Autodesk Fusion 360 part; units mm, degrees
(part 3 of 4)
  spline S294 degree 3 poles (-68.0103, -62.366) (-67.2714, -61.5215) (-66.1636, -61.0119) (-65.0416, -61.0002) (-63.8919, -60.9883) (-62.7469, -61.5006) (-61.9897, -62.366) knots -1 -1 -1 -1 -0.506107 -0.506107 -0.506107 0 0 0 0
  spline S295 degree 3 poles (-61.9897, -62.366) (-61.3663, -63.0785) (-61.0085, -64.0182) (-61.0002, -64.9649) (-60.9916, -65.935) (-61.3508, -66.9039) (-61.9897, -67.634) knots -1 -1 -1 -1 -0.506107 -0.506107 -0.506107 0 0 0 0
  spline S296 degree 3 poles (-61.9897, -57.634) (-62.7286, -58.4785) (-63.8364, -58.9881) (-64.9584, -58.9998) (-66.1081, -59.0117) (-67.2531, -58.4994) (-68.0103, -57.634) knots -1 -1 -1 -1 -0.506107 -0.506107 -0.506107 0 0 0 0
  spline S297 degree 3 poles (-68.0103, -57.634) (-68.6337, -56.9215) (-68.9915, -55.9818) (-68.9998, -55.0351) (-69.0084, -54.065) (-68.6492, -53.0961) (-68.0103, -52.366) knots -1 -1 -1 -1 -0.506107 -0.506107 -0.506107 0 0 0 0
  spline S298 degree 3 poles (-68.0103, -52.366) (-67.2714, -51.5215) (-66.1636, -51.0119) (-65.0416, -51.0002) (-63.8919, -50.9883) (-62.7469, -51.5006) (-61.9897, -52.366) knots -1 -1 -1 -1 -0.506107 -0.506107 -0.506107 0 0 0 0
  spline S299 degree 3 poles (-61.9897, -52.366) (-61.3663, -53.0785) (-61.0085, -54.0182) (-61.0002, -54.9649) (-60.9916, -55.935) (-61.3508, -56.9039) (-61.9897, -57.634) knots -1 -1 -1 -1 -0.506107 -0.506107 -0.506107 0 0 0 0
  spline S300 degree 3 poles (-61.9897, -47.634) (-62.7286, -48.4785) (-63.8364, -48.9881) (-64.9584, -48.9998) (-66.1081, -49.0117) (-67.2531, -48.4994) (-68.0103, -47.634) knots -1 -1 -1 -1 -0.506107 -0.506107 -0.506107 0 0 0 0
  spline S301 degree 3 poles (-68.0103, -47.634) (-68.6337, -46.9215) (-68.9915, -45.9818) (-68.9998, -45.0351) (-69.0084, -44.065) (-68.6492, -43.0961) (-68.0103, -42.366) knots -1 -1 -1 -1 -0.506107 -0.506107 -0.506107 0 0 0 0
  spline S302 degree 3 poles (-68.0103, -42.366) (-67.2714, -41.5215) (-66.1636, -41.0119) (-65.0416, -41.0002) (-63.8919, -40.9883) (-62.7469, -41.5006) (-61.9897, -42.366) knots -1 -1 -1 -1 -0.506107 -0.506107 -0.506107 0 0 0 0
  spline S303 degree 3 poles (-61.9897, -42.366) (-61.3663, -43.0785) (-61.0085, -44.0182) (-61.0002, -44.9649) (-60.9916, -45.935) (-61.3508, -46.9039) (-61.9897, -47.634) knots -1 -1 -1 -1 -0.506107 -0.506107 -0.506107 0 0 0 0
  spline S304 degree 3 poles (-61.9897, -37.634) (-62.7286, -38.4785) (-63.8364, -38.9881) (-64.9584, -38.9998) (-66.1081, -39.0117) (-67.2531, -38.4994) (-68.0103, -37.634) knots -1 -1 -1 -1 -0.506107 -0.506107 -0.506107 0 0 0 0
  spline S305 degree 3 poles (-68.0103, -37.634) (-68.6337, -36.9215) (-68.9915, -35.9818) (-68.9998, -35.0351) (-69.0084, -34.065) (-68.6492, -33.0961) (-68.0103, -32.366) knots -1 -1 -1 -1 -0.506107 -0.506107 -0.506107 0 0 0 0
  spline S306 degree 3 poles (-68.0103, -32.366) (-67.2714, -31.5215) (-66.1636, -31.0119) (-65.0416, -31.0002) (-63.8919, -30.9883) (-62.7469, -31.5006) (-61.9897, -32.366) knots -1 -1 -1 -1 -0.506107 -0.506107 -0.506107 0 0 0 0
  spline S307 degree 3 poles (-61.9897, -32.366) (-61.3663, -33.0785) (-61.0085, -34.0182) (-61.0002, -34.9649) (-60.9916, -35.935) (-61.3508, -36.9039) (-61.9897, -37.634) knots -1 -1 -1 -1 -0.506107 -0.506107 -0.506107 0 0 0 0
  spline S308 degree 3 poles (-61.9897, -27.634) (-62.7286, -28.4785) (-63.8364, -28.9881) (-64.9584, -28.9998) (-66.1081, -29.0117) (-67.2531, -28.4994) (-68.0103, -27.634) knots -1 -1 -1 -1 -0.506107 -0.506107 -0.506107 0 0 0 0
  spline S309 degree 3 poles (-68.0103, -27.634) (-68.6337, -26.9215) (-68.9915, -25.9818) (-68.9998, -25.0351) (-69.0084, -24.065) (-68.6492, -23.0961) (-68.0103, -22.366) knots -1 -1 -1 -1 -0.506107 -0.506107 -0.506107 0 0 0 0
  spline S310 degree 3 poles (-68.0103, -22.366) (-67.2714, -21.5215) (-66.1636, -21.0119) (-65.0416, -21.0002) (-63.8919, -20.9883) (-62.7469, -21.5006) (-61.9897, -22.366) knots -1 -1 -1 -1 -0.506107 -0.506107 -0.506107 0 0 0 0
  spline S311 degree 3 poles (-61.9897, -22.366) (-61.3663, -23.0785) (-61.0085, -24.0182) (-61.0002, -24.9649) (-60.9916, -25.935) (-61.3508, -26.9039) (-61.9897, -27.634) knots -1 -1 -1 -1 -0.506107 -0.506107 -0.506107 0 0 0 0
  spline S312 degree 3 poles (-61.9897, -17.634) (-62.7286, -18.4785) (-63.8364, -18.9881) (-64.9584, -18.9998) (-66.1081, -19.0117) (-67.2531, -18.4994) (-68.0103, -17.634) knots -1 -1 -1 -1 -0.506107 -0.506107 -0.506107 0 0 0 0
  spline S313 degree 3 poles (-68.0103, -17.634) (-68.6337, -16.9215) (-68.9915, -15.9818) (-68.9998, -15.0351) (-69.0084, -14.065) (-68.6492, -13.0961) (-68.0103, -12.366) knots -1 -1 -1 -1 -0.506107 -0.506107 -0.506107 0 0 0 0
  spline S314 degree 3 poles (-68.0103, -12.366) (-67.2714, -11.5215) (-66.1636, -11.0119) (-65.0416, -11.0002) (-63.8919, -10.9883) (-62.7469, -11.5006) (-61.9897, -12.366) knots -1 -1 -1 -1 -0.506107 -0.506107 -0.506107 0 0 0 0
  spline S315 degree 3 poles (-61.9897, -12.366) (-61.3663, -13.0785) (-61.0085, -14.0182) (-61.0002, -14.9649) (-60.9916, -15.935) (-61.3508, -16.9039) (-61.9897, -17.634) knots -1 -1 -1 -1 -0.506107 -0.506107 -0.506107 0 0 0 0
  spline S316 degree 3 poles (-61.9897, -7.634) (-62.7286, -8.4785) (-63.8364, -8.9881) (-64.9584, -8.9998) (-66.1081, -9.0117) (-67.2531, -8.4994) (-68.0103, -7.634) knots -1 -1 -1 -1 -0.506107 -0.506107 -0.506107 0 0 0 0
  spline S317 degree 3 poles (-68.0103, -7.634) (-68.6337, -6.9215) (-68.9915, -5.9818) (-68.9998, -5.0351) (-69.0084, -4.065) (-68.6492, -3.0961) (-68.0103, -2.366) knots -1 -1 -1 -1 -0.506107 -0.506107 -0.506107 0 0 0 0
  spline S318 degree 3 poles (-68.0103, -2.366) (-67.2714, -1.5215) (-66.1636, -1.0119) (-65.0416, -1.0002) (-63.8919, -0.9883) (-62.7469, -1.5006) (-61.9897, -2.366) knots -1 -1 -1 -1 -0.506107 -0.506107 -0.506107 0 0 0 0
  spline S319 degree 3 poles (-61.9897, -2.366) (-61.3663, -3.0785) (-61.0085, -4.0182) (-61.0002, -4.9649) (-60.9916, -5.935) (-61.3508, -6.9039) (-61.9897, -7.634) knots -1 -1 -1 -1 -0.506107 -0.506107 -0.506107 0 0 0 0
  spline S320 degree 3 poles (-51.9897, -77.634) (-52.7286, -78.4785) (-53.8364, -78.9881) (-54.9584, -78.9998) (-56.1081, -79.0117) (-57.2531, -78.4994) (-58.0103, -77.634) knots -1 -1 -1 -1 -0.506107 -0.506107 -0.506107 0 0 0 0
  spline S321 degree 3 poles (-58.0103, -77.634) (-58.6337, -76.9215) (-58.9915, -75.9818) (-58.9998, -75.0351) (-59.0084, -74.065) (-58.6492, -73.0961) (-58.0103, -72.366) knots -1 -1 -1 -1 -0.506107 -0.506107 -0.506107 0 0 0 0
  spline S322 degree 3 poles (-58.0103, -72.366) (-57.2714, -71.5215) (-56.1636, -71.0119) (-55.0416, -71.0002) (-53.8919, -70.9883) (-52.7469, -71.5006) (-51.9897, -72.366) knots -1 -1 -1 -1 -0.506107 -0.506107 -0.506107 0 0 0 0
  spline S323 degree 3 poles (-51.9897, -72.366) (-51.3663, -73.0785) (-51.0085, -74.0182) (-51.0002, -74.9649) (-50.9916, -75.935) (-51.3508, -76.9039) (-51.9897, -77.634) knots -1 -1 -1 -1 -0.506107 -0.506107 -0.506107 0 0 0 0
  spline S324 degree 3 poles (-51.9897, -67.634) (-52.7286, -68.4785) (-53.8364, -68.9881) (-54.9584, -68.9998) (-56.1081, -69.0117) (-57.2531, -68.4994) (-58.0103, -67.634) knots -1 -1 -1 -1 -0.506107 -0.506107 -0.506107 0 0 0 0
  spline S325 degree 3 poles (-58.0103, -67.634) (-58.6337, -66.9215) (-58.9915, -65.9818) (-58.9998, -65.0351) (-59.0084, -64.065) (-58.6492, -63.0961) (-58.0103, -62.366) knots -1 -1 -1 -1 -0.506107 -0.506107 -0.506107 0 0 0 0
  spline S326 degree 3 poles (-58.0103, -62.366) (-57.2714, -61.5215) (-56.1636, -61.0119) (-55.0416, -61.0002) (-53.8919, -60.9883) (-52.7469, -61.5006) (-51.9897, -62.366) knots -1 -1 -1 -1 -0.506107 -0.506107 -0.506107 0 0 0 0
  spline S327 degree 3 poles (-51.9897, -62.366) (-51.3663, -63.0785) (-51.0085, -64.0182) (-51.0002, -64.9649) (-50.9916, -65.935) (-51.3508, -66.9039) (-51.9897, -67.634) knots -1 -1 -1 -1 -0.506107 -0.506107 -0.506107 0 0 0 0
  spline S328 degree 3 poles (-51.9897, -57.634) (-52.7286, -58.4785) (-53.8364, -58.9881) (-54.9584, -58.9998) (-56.1081, -59.0117) (-57.2531, -58.4994) (-58.0103, -57.634) knots -1 -1 -1 -1 -0.506107 -0.506107 -0.506107 0 0 0 0
  spline S329 degree 3 poles (-58.0103, -57.634) (-58.6337, -56.9215) (-58.9915, -55.9818) (-58.9998, -55.0351) (-59.0084, -54.065) (-58.6492, -53.0961) (-58.0103, -52.366) knots -1 -1 -1 -1 -0.506107 -0.506107 -0.506107 0 0 0 0
  spline S330 degree 3 poles (-58.0103, -52.366) (-57.2714, -51.5215) (-56.1636, -51.0119) (-55.0416, -51.0002) (-53.8919, -50.9883) (-52.7469, -51.5006) (-51.9897, -52.366) knots -1 -1 -1 -1 -0.506107 -0.506107 -0.506107 0 0 0 0
  spline S331 degree 3 poles (-51.9897, -52.366) (-51.3663, -53.0785) (-51.0085, -54.0182) (-51.0002, -54.9649) (-50.9916, -55.935) (-51.3508, -56.9039) (-51.9897, -57.634) knots -1 -1 -1 -1 -0.506107 -0.506107 -0.506107 0 0 0 0
  spline S332 degree 3 poles (-51.9897, -47.634) (-52.7286, -48.4785) (-53.8364, -48.9881) (-54.9584, -48.9998) (-56.1081, -49.0117) (-57.2531, -48.4994) (-58.0103, -47.634) knots -1 -1 -1 -1 -0.506107 -0.506107 -0.506107 0 0 0 0
  spline S333 degree 3 poles (-58.0103, -47.634) (-58.6337, -46.9215) (-58.9915, -45.9818) (-58.9998, -45.0351) (-59.0084, -44.065) (-58.6492, -43.0961) (-58.0103, -42.366) knots -1 -1 -1 -1 -0.506107 -0.506107 -0.506107 0 0 0 0
  spline S334 degree 3 poles (-58.0103, -42.366) (-57.2714, -41.5215) (-56.1636, -41.0119) (-55.0416, -41.0002) (-53.8919, -40.9883) (-52.7469, -41.5006) (-51.9897, -42.366) knots -1 -1 -1 -1 -0.506107 -0.506107 -0.506107 0 0 0 0
  spline S335 degree 3 poles (-51.9897, -42.366) (-51.3663, -43.0785) (-51.0085, -44.0182) (-51.0002, -44.9649) (-50.9916, -45.935) (-51.3508, -46.9039) (-51.9897, -47.634) knots -1 -1 -1 -1 -0.506107 -0.506107 -0.506107 0 0 0 0
  spline S336 degree 3 poles (-51.9897, -37.634) (-52.7286, -38.4785) (-53.8364, -38.9881) (-54.9584, -38.9998) (-56.1081, -39.0117) (-57.2531, -38.4994) (-58.0103, -37.634) knots -1 -1 -1 -1 -0.506107 -0.506107 -0.506107 0 0 0 0
  spline S337 degree 3 poles (-58.0103, -37.634) (-58.6337, -36.9215) (-58.9915, -35.9818) (-58.9998, -35.0351) (-59.0084, -34.065) (-58.6492, -33.0961) (-58.0103, -32.366) knots -1 -1 -1 -1 -0.506107 -0.506107 -0.506107 0 0 0 0
  spline S338 degree 3 poles (-58.0103, -32.366) (-57.2714, -31.5215) (-56.1636, -31.0119) (-55.0416, -31.0002) (-53.8919, -30.9883) (-52.7469, -31.5006) (-51.9897, -32.366) knots -1 -1 -1 -1 -0.506107 -0.506107 -0.506107 0 0 0 0
  spline S339 degree 3 poles (-51.9897, -32.366) (-51.3663, -33.0785) (-51.0085, -34.0182) (-51.0002, -34.9649) (-50.9916, -35.935) (-51.3508, -36.9039) (-51.9897, -37.634) knots -1 -1 -1 -1 -0.506107 -0.506107 -0.506107 0 0 0 0
  spline S340 degree 3 poles (-51.9897, -27.634) (-52.7286, -28.4785) (-53.8364, -28.9881) (-54.9584, -28.9998) (-56.1081, -29.0117) (-57.2531, -28.4994) (-58.0103, -27.634) knots -1 -1 -1 -1 -0.506107 -0.506107 -0.506107 0 0 0 0
  spline S341 degree 3 poles (-58.0103, -27.634) (-58.6337, -26.9215) (-58.9915, -25.9818) (-58.9998, -25.0351) (-59.0084, -24.065) (-58.6492, -23.0961) (-58.0103, -22.366) knots -1 -1 -1 -1 -0.506107 -0.506107 -0.506107 0 0 0 0
  spline S342 degree 3 poles (-58.0103, -22.366) (-57.2714, -21.5215) (-56.1636, -21.0119) (-55.0416, -21.0002) (-53.8919, -20.9883) (-52.7469, -21.5006) (-51.9897, -22.366) knots -1 -1 -1 -1 -0.506107 -0.506107 -0.506107 0 0 0 0
  spline S343 degree 3 poles (-51.9897, -22.366) (-51.3663, -23.0785) (-51.0085, -24.0182) (-51.0002, -24.9649) (-50.9916, -25.935) (-51.3508, -26.9039) (-51.9897, -27.634) knots -1 -1 -1 -1 -0.506107 -0.506107 -0.506107 0 0 0 0
  spline S344 degree 3 poles (-51.9897, -17.634) (-52.7286, -18.4785) (-53.8364, -18.9881) (-54.9584, -18.9998) (-56.1081, -19.0117) (-57.2531, -18.4994) (-58.0103, -17.634) knots -1 -1 -1 -1 -0.506107 -0.506107 -0.506107 0 0 0 0
  spline S345 degree 3 poles (-58.0103, -17.634) (-58.6337, -16.9215) (-58.9915, -15.9818) (-58.9998, -15.0351) (-59.0084, -14.065) (-58.6492, -13.0961) (-58.0103, -12.366) knots -1 -1 -1 -1 -0.506107 -0.506107 -0.506107 0 0 0 0
  spline S346 degree 3 poles (-58.0103, -12.366) (-57.2714, -11.5215) (-56.1636, -11.0119) (-55.0416, -11.0002) (-53.8919, -10.9883) (-52.7469, -11.5006) (-51.9897, -12.366) knots -1 -1 -1 -1 -0.506107 -0.506107 -0.506107 0 0 0 0
  spline S347 degree 3 poles (-51.9897, -12.366) (-51.3663, -13.0785) (-51.0085, -14.0182) (-51.0002, -14.9649) (-50.9916, -15.935) (-51.3508, -16.9039) (-51.9897, -17.634) knots -1 -1 -1 -1 -0.506107 -0.506107 -0.506107 0 0 0 0
  spline S348 degree 3 poles (-51.9897, -7.634) (-52.7286, -8.4785) (-53.8364, -8.9881) (-54.9584, -8.9998) (-56.1081, -9.0117) (-57.2531, -8.4994) (-58.0103, -7.634) knots -1 -1 -1 -1 -0.506107 -0.506107 -0.506107 0 0 0 0
  spline S349 degree 3 poles (-58.0103, -7.634) (-58.6337, -6.9215) (-58.9915, -5.9818) (-58.9998, -5.0351) (-59.0084, -4.065) (-58.6492, -3.0961) (-58.0103, -2.366) knots -1 -1 -1 -1 -0.506107 -0.506107 -0.506107 0 0 0 0
  spline S350 degree 3 poles (-58.0103, -2.366) (-57.2714, -1.5215) (-56.1636, -1.0119) (-55.0416, -1.0002) (-53.8919, -0.9883) (-52.7469, -1.5006) (-51.9897, -2.366) knots -1 -1 -1 -1 -0.506107 -0.506107 -0.506107 0 0 0 0
  spline S351 degree 3 poles (-51.9897, -2.366) (-51.3663, -3.0785) (-51.0085, -4.0182) (-51.0002, -4.9649) (-50.9916, -5.935) (-51.3508, -6.9039) (-51.9897, -7.634) knots -1 -1 -1 -1 -0.506107 -0.506107 -0.506107 0 0 0 0
  spline S352 degree 3 poles (-41.9897, -77.634) (-42.7286, -78.4785) (-43.8364, -78.9881) (-44.9584, -78.9998) (-46.1081, -79.0117) (-47.2531, -78.4994) (-48.0103, -77.634) knots -1 -1 -1 -1 -0.506107 -0.506107 -0.506107 0 0 0 0
  spline S353 degree 3 poles (-48.0103, -77.634) (-48.6337, -76.9215) (-48.9915, -75.9818) (-48.9998, -75.0351) (-49.0084, -74.065) (-48.6492, -73.0961) (-48.0103, -72.366) knots -1 -1 -1 -1 -0.506107 -0.506107 -0.506107 0 0 0 0
  spline S354 degree 3 poles (-48.0103, -72.366) (-47.2714, -71.5215) (-46.1636, -71.0119) (-45.0416, -71.0002) (-43.8919, -70.9883) (-42.7469, -71.5006) (-41.9897, -72.366) knots -1 -1 -1 -1 -0.506107 -0.506107 -0.506107 0 0 0 0
  spline S355 degree 3 poles (-41.9897, -72.366) (-41.3663, -73.0785) (-41.0085, -74.0182) (-41.0002, -74.9649) (-40.9916, -75.935) (-41.3508, -76.9039) (-41.9897, -77.634) knots -1 -1 -1 -1 -0.506107 -0.506107 -0.506107 0 0 0 0
  spline S356 degree 3 poles (-41.9897, -67.634) (-42.7286, -68.4785) (-43.8364, -68.9881) (-44.9584, -68.9998) (-46.1081, -69.0117) (-47.2531, -68.4994) (-48.0103, -67.634) knots -1 -1 -1 -1 -0.506107 -0.506107 -0.506107 0 0 0 0
  spline S357 degree 3 poles (-48.0103, -67.634) (-48.6337, -66.9215) (-48.9915, -65.9818) (-48.9998, -65.0351) (-49.0084, -64.065) (-48.6492, -63.0961) (-48.0103, -62.366) knots -1 -1 -1 -1 -0.506107 -0.506107 -0.506107 0 0 0 0
  spline S358 degree 3 poles (-48.0103, -62.366) (-47.2714, -61.5215) (-46.1636, -61.0119) (-45.0416, -61.0002) (-43.8919, -60.9883) (-42.7469, -61.5006) (-41.9897, -62.366) knots -1 -1 -1 -1 -0.506107 -0.506107 -0.506107 0 0 0 0
  spline S359 degree 3 poles (-41.9897, -62.366) (-41.3663, -63.0785) (-41.0085, -64.0182) (-41.0002, -64.9649) (-40.9916, -65.935) (-41.3508, -66.9039) (-41.9897, -67.634) knots -1 -1 -1 -1 -0.506107 -0.506107 -0.506107 0 0 0 0
  spline S360 degree 3 poles (-41.9897, -57.634) (-42.7286, -58.4785) (-43.8364, -58.9881) (-44.9584, -58.9998) (-46.1081, -59.0117) (-47.2531, -58.4994) (-48.0103, -57.634) knots -1 -1 -1 -1 -0.506107 -0.506107 -0.506107 0 0 0 0
  spline S361 degree 3 poles (-48.0103, -57.634) (-48.6337, -56.9215) (-48.9915, -55.9818) (-48.9998, -55.0351) (-49.0084, -54.065) (-48.6492, -53.0961) (-48.0103, -52.366) knots -1 -1 -1 -1 -0.506107 -0.506107 -0.506107 0 0 0 0
  spline S362 degree 3 poles (-48.0103, -52.366) (-47.2714, -51.5215) (-46.1636, -51.0119) (-45.0416, -51.0002) (-43.8919, -50.9883) (-42.7469, -51.5006) (-41.9897, -52.366) knots -1 -1 -1 -1 -0.506107 -0.506107 -0.506107 0 0 0 0
  spline S363 degree 3 poles (-41.9897, -52.366) (-41.3663, -53.0785) (-41.0085, -54.0182) (-41.0002, -54.9649) (-40.9916, -55.935) (-41.3508, -56.9039) (-41.9897, -57.634) knots -1 -1 -1 -1 -0.506107 -0.506107 -0.506107 0 0 0 0
  spline S364 degree 3 poles (-41.9897, -47.634) (-42.7286, -48.4785) (-43.8364, -48.9881) (-44.9584, -48.9998) (-46.1081, -49.0117) (-47.2531, -48.4994) (-48.0103, -47.634) knots -1 -1 -1 -1 -0.506107 -0.506107 -0.506107 0 0 0 0
  spline S365 degree 3 poles (-48.0103, -47.634) (-48.6337, -46.9215) (-48.9915, -45.9818) (-48.9998, -45.0351) (-49.0084, -44.065) (-48.6492, -43.0961) (-48.0103, -42.366) knots -1 -1 -1 -1 -0.506107 -0.506107 -0.506107 0 0 0 0
  spline S366 degree 3 poles (-48.0103, -42.366) (-47.2714, -41.5215) (-46.1636, -41.0119) (-45.0416, -41.0002) (-43.8919, -40.9883) (-42.7469, -41.5006) (-41.9897, -42.366) knots -1 -1 -1 -1 -0.506107 -0.506107 -0.506107 0 0 0 0
  spline S367 degree 3 poles (-41.9897, -42.366) (-41.3663, -43.0785) (-41.0085, -44.0182) (-41.0002, -44.9649) (-40.9916, -45.935) (-41.3508, -46.9039) (-41.9897, -47.634) knots -1 -1 -1 -1 -0.506107 -0.506107 -0.506107 0 0 0 0
  spline S368 degree 3 poles (-41.9897, -37.634) (-42.7286, -38.4785) (-43.8364, -38.9881) (-44.9584, -38.9998) (-46.1081, -39.0117) (-47.2531, -38.4994) (-48.0103, -37.634) knots -1 -1 -1 -1 -0.506107 -0.506107 -0.506107 0 0 0 0
  spline S369 degree 3 poles (-48.0103, -37.634) (-48.6337, -36.9215) (-48.9915, -35.9818) (-48.9998, -35.0351) (-49.0084, -34.065) (-48.6492, -33.0961) (-48.0103, -32.366) knots -1 -1 -1 -1 -0.506107 -0.506107 -0.506107 0 0 0 0
  spline S370 degree 3 poles (-48.0103, -32.366) (-47.2714, -31.5215) (-46.1636, -31.0119) (-45.0416, -31.0002) (-43.8919, -30.9883) (-42.7469, -31.5006) (-41.9897, -32.366) knots -1 -1 -1 -1 -0.506107 -0.506107 -0.506107 0 0 0 0
  spline S371 degree 3 poles (-41.9897, -32.366) (-41.3663, -33.0785) (-41.0085, -34.0182) (-41.0002, -34.9649) (-40.9916, -35.935) (-41.3508, -36.9039) (-41.9897, -37.634) knots -1 -1 -1 -1 -0.506107 -0.506107 -0.506107 0 0 0 0
  spline S372 degree 3 poles (-41.9897, -27.634) (-42.7286, -28.4785) (-43.8364, -28.9881) (-44.9584, -28.9998) (-46.1081, -29.0117) (-47.2531, -28.4994) (-48.0103, -27.634) knots -1 -1 -1 -1 -0.506107 -0.506107 -0.506107 0 0 0 0
  spline S373 degree 3 poles (-48.0103, -27.634) (-48.6337, -26.9215) (-48.9915, -25.9818) (-48.9998, -25.0351) (-49.0084, -24.065) (-48.6492, -23.0961) (-48.0103, -22.366) knots -1 -1 -1 -1 -0.506107 -0.506107 -0.506107 0 0 0 0
  spline S374 degree 3 poles (-48.0103, -22.366) (-47.2714, -21.5215) (-46.1636, -21.0119) (-45.0416, -21.0002) (-43.8919, -20.9883) (-42.7469, -21.5006) (-41.9897, -22.366) knots -1 -1 -1 -1 -0.506107 -0.506107 -0.506107 0 0 0 0
  spline S375 degree 3 poles (-41.9897, -22.366) (-41.3663, -23.0785) (-41.0085, -24.0182) (-41.0002, -24.9649) (-40.9916, -25.935) (-41.3508, -26.9039) (-41.9897, -27.634) knots -1 -1 -1 -1 -0.506107 -0.506107 -0.506107 0 0 0 0
  spline S376 degree 3 poles (-41.9897, -17.634) (-42.7286, -18.4785) (-43.8364, -18.9881) (-44.9584, -18.9998) (-46.1081, -19.0117) (-47.2531, -18.4994) (-48.0103, -17.634) knots -1 -1 -1 -1 -0.506107 -0.506107 -0.506107 0 0 0 0
  spline S377 degree 3 poles (-48.0103, -17.634) (-48.6337, -16.9215) (-48.9915, -15.9818) (-48.9998, -15.0351) (-49.0084, -14.065) (-48.6492, -13.0961) (-48.0103, -12.366) knots -1 -1 -1 -1 -0.506107 -0.506107 -0.506107 0 0 0 0
  spline S378 degree 3 poles (-48.0103, -12.366) (-47.2714, -11.5215) (-46.1636, -11.0119) (-45.0416, -11.0002) (-43.8919, -10.9883) (-42.7469, -11.5006) (-41.9897, -12.366) knots -1 -1 -1 -1 -0.506107 -0.506107 -0.506107 0 0 0 0
  spline S379 degree 3 poles (-41.9897, -12.366) (-41.3663, -13.0785) (-41.0085, -14.0182) (-41.0002, -14.9649) (-40.9916, -15.935) (-41.3508, -16.9039) (-41.9897, -17.634) knots -1 -1 -1 -1 -0.506107 -0.506107 -0.506107 0 0 0 0
  spline S380 degree 3 poles (-41.9897, -7.634) (-42.7286, -8.4785) (-43.8364, -8.9881) (-44.9584, -8.9998) (-46.1081, -9.0117) (-47.2531, -8.4994) (-48.0103, -7.634) knots -1 -1 -1 -1 -0.506107 -0.506107 -0.506107 0 0 0 0
  spline S381 degree 3 poles (-48.0103, -7.634) (-48.6337, -6.9215) (-48.9915, -5.9818) (-48.9998, -5.0351) (-49.0084, -4.065) (-48.6492, -3.0961) (-48.0103, -2.366) knots -1 -1 -1 -1 -0.506107 -0.506107 -0.506107 0 0 0 0
  spline S382 degree 3 poles (-48.0103, -2.366) (-47.2714, -1.5215) (-46.1636, -1.0119) (-45.0416, -1.0002) (-43.8919, -0.9883) (-42.7469, -1.5006) (-41.9897, -2.366) knots -1 -1 -1 -1 -0.506107 -0.506107 -0.506107 0 0 0 0
  spline S383 degree 3 poles (-41.9897, -2.366) (-41.3663, -3.0785) (-41.0085, -4.0182) (-41.0002, -4.9649) (-40.9916, -5.935) (-41.3508, -6.9039) (-41.9897, -7.634) knots -1 -1 -1 -1 -0.506107 -0.506107 -0.506107 0 0 0 0
  spline S384 degree 3 poles (-31.9897, -77.634) (-32.7286, -78.4785) (-33.8364, -78.9881) (-34.9584, -78.9998) (-36.1081, -79.0117) (-37.2531, -78.4994) (-38.0103, -77.634) knots -1 -1 -1 -1 -0.506107 -0.506107 -0.506107 0 0 0 0
  spline S385 degree 3 poles (-38.0103, -77.634) (-38.6337, -76.9215) (-38.9915, -75.9818) (-38.9998, -75.0351) (-39.0084, -74.065) (-38.6492, -73.0961) (-38.0103, -72.366) knots -1 -1 -1 -1 -0.506107 -0.506107 -0.506107 0 0 0 0
  spline S386 degree 3 poles (-38.0103, -72.366) (-37.2714, -71.5215) (-36.1636, -71.0119) (-35.0416, -71.0002) (-33.8919, -70.9883) (-32.7469, -71.5006) (-31.9897, -72.366) knots -1 -1 -1 -1 -0.506107 -0.506107 -0.506107 0 0 0 0
  spline S387 degree 3 poles (-31.9897, -72.366) (-31.3663, -73.0785) (-31.0085, -74.0182) (-31.0002, -74.9649) (-30.9916, -75.935) (-31.3508, -76.9039) (-31.9897, -77.634) knots -1 -1 -1 -1 -0.506107 -0.506107 -0.506107 0 0 0 0
  spline S388 degree 3 poles (-31.9897, -67.634) (-32.7286, -68.4785) (-33.8364, -68.9881) (-34.9584, -68.9998) (-36.1081, -69.0117) (-37.2531, -68.4994) (-38.0103, -67.634) knots -1 -1 -1 -1 -0.506107 -0.506107 -0.506107 0 0 0 0
  spline S389 degree 3 poles (-38.0103, -67.634) (-38.6337, -66.9215) (-38.9915, -65.9818) (-38.9998, -65.0351) (-39.0084, -64.065) (-38.6492, -63.0961) (-38.0103, -62.366) knots -1 -1 -1 -1 -0.506107 -0.506107 -0.506107 0 0 0 0
  spline S390 degree 3 poles (-38.0103, -62.366) (-37.2714, -61.5215) (-36.1636, -61.0119) (-35.0416, -61.0002) (-33.8919, -60.9883) (-32.7469, -61.5006) (-31.9897, -62.366) knots -1 -1 -1 -1 -0.506107 -0.506107 -0.506107 0 0 0 0
  spline S391 degree 3 poles (-31.9897, -62.366) (-31.3663, -63.0785) (-31.0085, -64.0182) (-31.0002, -64.9649) (-30.9916, -65.935) (-31.3508, -66.9039) (-31.9897, -67.634) knots -1 -1 -1 -1 -0.506107 -0.506107 -0.506107 0 0 0 0
  spline S392 degree 3 poles (-31.9897, -57.634) (-32.7286, -58.4785) (-33.8364, -58.9881) (-34.9584, -58.9998) (-36.1081, -59.0117) (-37.2531, -58.4994) (-38.0103, -57.634) knots -1 -1 -1 -1 -0.506107 -0.506107 -0.506107 0 0 0 0
  spline S393 degree 3 poles (-38.0103, -57.634) (-38.6337, -56.9215) (-38.9915, -55.9818) (-38.9998, -55.0351) (-39.0084, -54.065) (-38.6492, -53.0961) (-38.0103, -52.366) knots -1 -1 -1 -1 -0.506107 -0.506107 -0.506107 0 0 0 0
  spline S394 degree 3 poles (-38.0103, -52.366) (-37.2714, -51.5215) (-36.1636, -51.0119) (-35.0416, -51.0002) (-33.8919, -50.9883) (-32.7469, -51.5006) (-31.9897, -52.366) knots -1 -1 -1 -1 -0.506107 -0.506107 -0.506107 0 0 0 0
  spline S395 degree 3 poles (-31.9897, -52.366) (-31.3663, -53.0785) (-31.0085, -54.0182) (-31.0002, -54.9649) (-30.9916, -55.935) (-31.3508, -56.9039) (-31.9897, -57.634) knots -1 -1 -1 -1 -0.506107 -0.506107 -0.506107 0 0 0 0
  spline S396 degree 3 poles (-31.9897, -47.634) (-32.7286, -48.4785) (-33.8364, -48.9881) (-34.9584, -48.9998) (-36.1081, -49.0117) (-37.2531, -48.4994) (-38.0103, -47.634) knots -1 -1 -1 -1 -0.506107 -0.506107 -0.506107 0 0 0 0
  spline S397 degree 3 poles (-38.0103, -47.634) (-38.6337, -46.9215) (-38.9915, -45.9818) (-38.9998, -45.0351) (-39.0084, -44.065) (-38.6492, -43.0961) (-38.0103, -42.366) knots -1 -1 -1 -1 -0.506107 -0.506107 -0.506107 0 0 0 0
  spline S398 degree 3 poles (-38.0103, -42.366) (-37.2714, -41.5215) (-36.1636, -41.0119) (-35.0416, -41.0002) (-33.8919, -40.9883) (-32.7469, -41.5006) (-31.9897, -42.366) knots -1 -1 -1 -1 -0.506107 -0.506107 -0.506107 0 0 0 0
  spline S399 degree 3 poles (-31.9897, -42.366) (-31.3663, -43.0785) (-31.0085, -44.0182) (-31.0002, -44.9649) (-30.9916, -45.935) (-31.3508, -46.9039) (-31.9897, -47.634) knots -1 -1 -1 -1 -0.506107 -0.506107 -0.506107 0 0 0 0
  spline S400 degree 3 poles (-31.9897, -37.634) (-32.7286, -38.4785) (-33.8364, -38.9881) (-34.9584, -38.9998) (-36.1081, -39.0117) (-37.2531, -38.4994) (-38.0103, -37.634) knots -1 -1 -1 -1 -0.506107 -0.506107 -0.506107 0 0 0 0
  spline S401 degree 3 poles (-38.0103, -37.634) (-38.6337, -36.9215) (-38.9915, -35.9818) (-38.9998, -35.0351) (-39.0084, -34.065) (-38.6492, -33.0961) (-38.0103, -32.366) knots -1 -1 -1 -1 -0.506107 -0.506107 -0.506107 0 0 0 0
  spline S402 degree 3 poles (-38.0103, -32.366) (-37.2714, -31.5215) (-36.1636, -31.0119) (-35.0416, -31.0002) (-33.8919, -30.9883) (-32.7469, -31.5006) (-31.9897, -32.366) knots -1 -1 -1 -1 -0.506107 -0.506107 -0.506107 0 0 0 0
  spline S403 degree 3 poles (-31.9897, -32.366) (-31.3663, -33.0785) (-31.0085, -34.0182) (-31.0002, -34.9649) (-30.9916, -35.935) (-31.3508, -36.9039) (-31.9897, -37.634) knots -1 -1 -1 -1 -0.506107 -0.506107 -0.506107 0 0 0 0
  spline S404 degree 3 poles (-31.9897, -27.634) (-32.7286, -28.4785) (-33.8364, -28.9881) (-34.9584, -28.9998) (-36.1081, -29.0117) (-37.2531, -28.4994) (-38.0103, -27.634) knots -1 -1 -1 -1 -0.506107 -0.506107 -0.506107 0 0 0 0
  spline S405 degree 3 poles (-38.0103, -27.634) (-38.6337, -26.9215) (-38.9915, -25.9818) (-38.9998, -25.0351) (-39.0084, -24.065) (-38.6492, -23.0961) (-38.0103, -22.366) knots -1 -1 -1 -1 -0.506107 -0.506107 -0.506107 0 0 0 0
  spline S406 degree 3 poles (-38.0103, -22.366) (-37.2714, -21.5215) (-36.1636, -21.0119) (-35.0416, -21.0002) (-33.8919, -20.9883) (-32.7469, -21.5006) (-31.9897, -22.366) knots -1 -1 -1 -1 -0.506107 -0.506107 -0.506107 0 0 0 0
  spline S407 degree 3 poles (-31.9897, -22.366) (-31.3663, -23.0785) (-31.0085, -24.0182) (-31.0002, -24.9649) (-30.9916, -25.935) (-31.3508, -26.9039) (-31.9897, -27.634) knots -1 -1 -1 -1 -0.506107 -0.506107 -0.506107 0 0 0 0
  spline S408 degree 3 poles (-31.9897, -17.634) (-32.7286, -18.4785) (-33.8364, -18.9881) (-34.9584, -18.9998) (-36.1081, -19.0117) (-37.2531, -18.4994) (-38.0103, -17.634) knots -1 -1 -1 -1 -0.506107 -0.506107 -0.506107 0 0 0 0
  spline S409 degree 3 poles (-38.0103, -17.634) (-38.6337, -16.9215) (-38.9915, -15.9818) (-38.9998, -15.0351) (-39.0084, -14.065) (-38.6492, -13.0961) (-38.0103, -12.366) knots -1 -1 -1 -1 -0.506107 -0.506107 -0.506107 0 0 0 0
  spline S410 degree 3 poles (-38.0103, -12.366) (-37.2714, -11.5215) (-36.1636, -11.0119) (-35.0416, -11.0002) (-33.8919, -10.9883) (-32.7469, -11.5006) (-31.9897, -12.366) knots -1 -1 -1 -1 -0.506107 -0.506107 -0.506107 0 0 0 0
  spline S411 degree 3 poles (-31.9897, -12.366) (-31.3663, -13.0785) (-31.0085, -14.0182) (-31.0002, -14.9649) (-30.9916, -15.935) (-31.3508, -16.9039) (-31.9897, -17.634) knots -1 -1 -1 -1 -0.506107 -0.506107 -0.506107 0 0 0 0
  spline S412 degree 3 poles (-31.9897, -7.634) (-32.7286, -8.4785) (-33.8364, -8.9881) (-34.9584, -8.9998) (-36.1081, -9.0117) (-37.2531, -8.4994) (-38.0103, -7.634) knots -1 -1 -1 -1 -0.506107 -0.506107 -0.506107 0 0 0 0
  spline S413 degree 3 poles (-38.0103, -7.634) (-38.6337, -6.9215) (-38.9915, -5.9818) (-38.9998, -5.0351) (-39.0084, -4.065) (-38.6492, -3.0961) (-38.0103, -2.366) knots -1 -1 -1 -1 -0.506107 -0.506107 -0.506107 0 0 0 0
  spline S414 degree 3 poles (-38.0103, -2.366) (-37.2714, -1.5215) (-36.1636, -1.0119) (-35.0416, -1.0002) (-33.8919, -0.9883) (-32.7469, -1.5006) (-31.9897, -2.366) knots -1 -1 -1 -1 -0.506107 -0.506107 -0.506107 0 0 0 0
  spline S415 degree 3 poles (-31.9897, -2.366) (-31.3663, -3.0785) (-31.0085, -4.0182) (-31.0002, -4.9649) (-30.9916, -5.935) (-31.3508, -6.9039) (-31.9897, -7.634) knots -1 -1 -1 -1 -0.506107 -0.506107 -0.506107 0 0 0 0
  spline S416 degree 3 poles (-21.9897, -77.634) (-22.7286, -78.4785) (-23.8364, -78.9881) (-24.9584, -78.9998) (-26.1081, -79.0117) (-27.2531, -78.4994) (-28.0103, -77.634) knots -1 -1 -1 -1 -0.506107 -0.506107 -0.506107 0 0 0 0
  spline S417 degree 3 poles (-28.0103, -77.634) (-28.6337, -76.9215) (-28.9915, -75.9818) (-28.9998, -75.0351) (-29.0084, -74.065) (-28.6492, -73.0961) (-28.0103, -72.366) knots -1 -1 -1 -1 -0.506107 -0.506107 -0.506107 0 0 0 0
  spline S418 degree 3 poles (-28.0103, -72.366) (-27.2714, -71.5215) (-26.1636, -71.0119) (-25.0416, -71.0002) (-23.8919, -70.9883) (-22.7469, -71.5006) (-21.9897, -72.366) knots -1 -1 -1 -1 -0.506107 -0.506107 -0.506107 0 0 0 0
  spline S419 degree 3 poles (-21.9897, -72.366) (-21.3663, -73.0785) (-21.0085, -74.0182) (-21.0002, -74.9649) (-20.9916, -75.935) (-21.3508, -76.9039) (-21.9897, -77.634) knots -1 -1 -1 -1 -0.506107 -0.506107 -0.506107 0 0 0 0
  spline S420 degree 3 poles (-21.9897, -67.634) (-22.7286, -68.4785) (-23.8364, -68.9881) (-24.9584, -68.9998) (-26.1081, -69.0117) (-27.2531, -68.4994) (-28.0103, -67.634) knots -1 -1 -1 -1 -0.506107 -0.506107 -0.506107 0 0 0 0
  spline S421 degree 3 poles (-28.0103, -67.634) (-28.6337, -66.9215) (-28.9915, -65.9818) (-28.9998, -65.0351) (-29.0084, -64.065) (-28.6492, -63.0961) (-28.0103, -62.366) knots -1 -1 -1 -1 -0.506107 -0.506107 -0.506107 0 0 0 0
  spline S422 degree 3 poles (-28.0103, -62.366) (-27.2714, -61.5215) (-26.1636, -61.0119) (-25.0416, -61.0002) (-23.8919, -60.9883) (-22.7469, -61.5006) (-21.9897, -62.366) knots -1 -1 -1 -1 -0.506107 -0.506107 -0.506107 0 0 0 0
  spline S423 degree 3 poles (-21.9897, -62.366) (-21.3663, -63.0785) (-21.0085, -64.0182) (-21.0002, -64.9649) (-20.9916, -65.935) (-21.3508, -66.9039) (-21.9897, -67.634) knots -1 -1 -1 -1 -0.506107 -0.506107 -0.506107 0 0 0 0
  spline S424 degree 3 poles (-21.9897, -57.634) (-22.7286, -58.4785) (-23.8364, -58.9881) (-24.9584, -58.9998) (-26.1081, -59.0117) (-27.2531, -58.4994) (-28.0103, -57.634) knots -1 -1 -1 -1 -0.506107 -0.506107 -0.506107 0 0 0 0
  spline S425 degree 3 poles (-28.0103, -57.634) (-28.6337, -56.9215) (-28.9915, -55.9818) (-28.9998, -55.0351) (-29.0084, -54.065) (-28.6492, -53.0961) (-28.0103, -52.366) knots -1 -1 -1 -1 -0.506107 -0.506107 -0.506107 0 0 0 0
  spline S426 degree 3 poles (-28.0103, -52.366) (-27.2714, -51.5215) (-26.1636, -51.0119) (-25.0416, -51.0002) (-23.8919, -50.9883) (-22.7469, -51.5006) (-21.9897, -52.366) knots -1 -1 -1 -1 -0.506107 -0.506107 -0.506107 0 0 0 0
  spline S427 degree 3 poles (-21.9897, -52.366) (-21.3663, -53.0785) (-21.0085, -54.0182) (-21.0002, -54.9649) (-20.9916, -55.935) (-21.3508, -56.9039) (-21.9897, -57.634) knots -1 -1 -1 -1 -0.506107 -0.506107 -0.506107 0 0 0 0
  spline S428 degree 3 poles (-21.9897, -47.634) (-22.7286, -48.4785) (-23.8364, -48.9881) (-24.9584, -48.9998) (-26.1081, -49.0117) (-27.2531, -48.4994) (-28.0103, -47.634) knots -1 -1 -1 -1 -0.506107 -0.506107 -0.506107 0 0 0 0
  spline S429 degree 3 poles (-28.0103, -47.634) (-28.6337, -46.9215) (-28.9915, -45.9818) (-28.9998, -45.0351) (-29.0084, -44.065) (-28.6492, -43.0961) (-28.0103, -42.366) knots -1 -1 -1 -1 -0.506107 -0.506107 -0.506107 0 0 0 0
  spline S430 degree 3 poles (-28.0103, -42.366) (-27.2714, -41.5215) (-26.1636, -41.0119) (-25.0416, -41.0002) (-23.8919, -40.9883) (-22.7469, -41.5006) (-21.9897, -42.366) knots -1 -1 -1 -1 -0.506107 -0.506107 -0.506107 0 0 0 0
  spline S431 degree 3 poles (-21.9897, -42.366) (-21.3663, -43.0785) (-21.0085, -44.0182) (-21.0002, -44.9649) (-20.9916, -45.935) (-21.3508, -46.9039) (-21.9897, -47.634) knots -1 -1 -1 -1 -0.506107 -0.506107 -0.506107 0 0 0 0
  spline S432 degree 3 poles (-21.9897, -37.634) (-22.7286, -38.4785) (-23.8364, -38.9881) (-24.9584, -38.9998) (-26.1081, -39.0117) (-27.2531, -38.4994) (-28.0103, -37.634) knots -1 -1 -1 -1 -0.506107 -0.506107 -0.506107 0 0 0 0
  spline S433 degree 3 poles (-28.0103, -37.634) (-28.6337, -36.9215) (-28.9915, -35.9818) (-28.9998, -35.0351) (-29.0084, -34.065) (-28.6492, -33.0961) (-28.0103, -32.366) knots -1 -1 -1 -1 -0.506107 -0.506107 -0.506107 0 0 0 0
  spline S434 degree 3 poles (-28.0103, -32.366) (-27.2714, -31.5215) (-26.1636, -31.0119) (-25.0416, -31.0002) (-23.8919, -30.9883) (-22.7469, -31.5006) (-21.9897, -32.366) knots -1 -1 -1 -1 -0.506107 -0.506107 -0.506107 0 0 0 0
  spline S435 degree 3 poles (-21.9897, -32.366) (-21.3663, -33.0785) (-21.0085, -34.0182) (-21.0002, -34.9649) (-20.9916, -35.935) (-21.3508, -36.9039) (-21.9897, -37.634) knots -1 -1 -1 -1 -0.506107 -0.506107 -0.506107 0 0 0 0
  spline S436 degree 3 poles (-21.9897, -27.634) (-22.7286, -28.4785) (-23.8364, -28.9881) (-24.9584, -28.9998) (-26.1081, -29.0117) (-27.2531, -28.4994) (-28.0103, -27.634) knots -1 -1 -1 -1 -0.506107 -0.506107 -0.506107 0 0 0 0
  spline S437 degree 3 poles (-28.0103, -27.634) (-28.6337, -26.9215) (-28.9915, -25.9818) (-28.9998, -25.0351) (-29.0084, -24.065) (-28.6492, -23.0961) (-28.0103, -22.366) knots -1 -1 -1 -1 -0.506107 -0.506107 -0.506107 0 0 0 0
  spline S438 degree 3 poles (-28.0103, -22.366) (-27.2714, -21.5215) (-26.1636, -21.0119) (-25.0416, -21.0002) (-23.8919, -20.9883) (-22.7469, -21.5006) (-21.9897, -22.366) knots -1 -1 -1 -1 -0.506107 -0.506107 -0.506107 0 0 0 0
  spline S439 degree 3 poles (-21.9897, -22.366) (-21.3663, -23.0785) (-21.0085, -24.0182) (-21.0002, -24.9649) (-20.9916, -25.935) (-21.3508, -26.9039) (-21.9897, -27.634) knots -1 -1 -1 -1 -0.506107 -0.506107 -0.506107 0 0 0 0
  spline S440 degree 3 poles (-21.9897, -17.634) (-22.7286, -18.4785) (-23.8364, -18.9881) (-24.9584, -18.9998) (-26.1081, -19.0117) (-27.2531, -18.4994) (-28.0103, -17.634) knots -1 -1 -1 -1 -0.506107 -0.506107 -0.506107 0 0 0 0
  spline S441 degree 3 poles (-28.0103, -17.634) (-28.6337, -16.9215) (-28.9915, -15.9818) (-28.9998, -15.0351) (-29.0084, -14.065) (-28.6492, -13.0961) (-28.0103, -12.366) knots -1 -1 -1 -1 -0.506107 -0.506107 -0.506107 0 0 0 0
  spline S442 degree 3 poles (-28.0103, -12.366) (-27.2714, -11.5215) (-26.1636, -11.0119) (-25.0416, -11.0002) (-23.8919, -10.9883) (-22.7469, -11.5006) (-21.9897, -12.366) knots -1 -1 -1 -1 -0.506107 -0.506107 -0.506107 0 0 0 0
  spline S443 degree 3 poles (-21.9897, -12.366) (-21.3663, -13.0785) (-21.0085, -14.0182) (-21.0002, -14.9649) (-20.9916, -15.935) (-21.3508, -16.9039) (-21.9897, -17.634) knots -1 -1 -1 -1 -0.506107 -0.506107 -0.506107 0 0 0 0
  spline S444 degree 3 poles (-21.9897, -7.634) (-22.7286, -8.4785) (-23.8364, -8.9881) (-24.9584, -8.9998) (-26.1081, -9.0117) (-27.2531, -8.4994) (-28.0103, -7.634) knots -1 -1 -1 -1 -0.506107 -0.506107 -0.506107 0 0 0 0
  spline S445 degree 3 poles (-28.0103, -7.634) (-28.6337, -6.9215) (-28.9915, -5.9818) (-28.9998, -5.0351) (-29.0084, -4.065) (-28.6492, -3.0961) (-28.0103, -2.366) knots -1 -1 -1 -1 -0.506107 -0.506107 -0.506107 0 0 0 0
  spline S446 degree 3 poles (-28.0103, -2.366) (-27.2714, -1.5215) (-26.1636, -1.0119) (-25.0416, -1.0002) (-23.8919, -0.9883) (-22.7469, -1.5006) (-21.9897, -2.366) knots -1 -1 -1 -1 -0.506107 -0.506107 -0.506107 0 0 0 0
  spline S447 degree 3 poles (-21.9897, -2.366) (-21.3663, -3.0785) (-21.0085, -4.0182) (-21.0002, -4.9649) (-20.9916, -5.935) (-21.3508, -6.9039) (-21.9897, -7.634) knots -1 -1 -1 -1 -0.506107 -0.506107 -0.506107 0 0 0 0
  spline S448 degree 3 poles (-11.9897, -77.634) (-12.7286, -78.4785) (-13.8364, -78.9881) (-14.9584, -78.9998) (-16.1081, -79.0117) (-17.2531, -78.4994) (-18.0103, -77.634) knots -1 -1 -1 -1 -0.506107 -0.506107 -0.506107 0 0 0 0
  spline S449 degree 3 poles (-18.0103, -77.634) (-18.6337, -76.9215) (-18.9915, -75.9818) (-18.9998, -75.0351) (-19.0084, -74.065) (-18.6492, -73.0961) (-18.0103, -72.366) knots -1 -1 -1 -1 -0.506107 -0.506107 -0.506107 0 0 0 0
  spline S450 degree 3 poles (-18.0103, -72.366) (-17.2714, -71.5215) (-16.1636, -71.0119) (-15.0416, -71.0002) (-13.8919, -70.9883) (-12.7469, -71.5006) (-11.9897, -72.366) knots -1 -1 -1 -1 -0.506107 -0.506107 -0.506107 0 0 0 0
  spline S451 degree 3 poles (-11.9897, -72.366) (-11.3663, -73.0785) (-11.0085, -74.0182) (-11.0002, -74.9649) (-10.9916, -75.935) (-11.3508, -76.9039) (-11.9897, -77.634) knots -1 -1 -1 -1 -0.506107 -0.506107 -0.506107 0 0 0 0
  spline S452 degree 3 poles (-11.9897, -67.634) (-12.7286, -68.4785) (-13.8364, -68.9881) (-14.9584, -68.9998) (-16.1081, -69.0117) (-17.2531, -68.4994) (-18.0103, -67.634) knots -1 -1 -1 -1 -0.506107 -0.506107 -0.506107 0 0 0 0
  spline S453 degree 3 poles (-18.0103, -67.634) (-18.6337, -66.9215) (-18.9915, -65.9818) (-18.9998, -65.0351) (-19.0084, -64.065) (-18.6492, -63.0961) (-18.0103, -62.366) knots -1 -1 -1 -1 -0.506107 -0.506107 -0.506107 0 0 0 0
  spline S454 degree 3 poles (-18.0103, -62.366) (-17.2714, -61.5215) (-16.1636, -61.0119) (-15.0416, -61.0002) (-13.8919, -60.9883) (-12.7469, -61.5006) (-11.9897, -62.366) knots -1 -1 -1 -1 -0.506107 -0.506107 -0.506107 0 0 0 0
  spline S455 degree 3 poles (-11.9897, -62.366) (-11.3663, -63.0785) (-11.0085, -64.0182) (-11.0002, -64.9649) (-10.9916, -65.935) (-11.3508, -66.9039) (-11.9897, -67.634) knots -1 -1 -1 -1 -0.506107 -0.506107 -0.506107 0 0 0 0
  spline S456 degree 3 poles (-11.9897, -57.634) (-12.7286, -58.4785) (-13.8364, -58.9881) (-14.9584, -58.9998) (-16.1081, -59.0117) (-17.2531, -58.4994) (-18.0103, -57.634) knots -1 -1 -1 -1 -0.506107 -0.506107 -0.506107 0 0 0 0
  spline S457 degree 3 poles (-18.0103, -57.634) (-18.6337, -56.9215) (-18.9915, -55.9818) (-18.9998, -55.0351) (-19.0084, -54.065) (-18.6492, -53.0961) (-18.0103, -52.366) knots -1 -1 -1 -1 -0.506107 -0.506107 -0.506107 0 0 0 0
  spline S458 degree 3 poles (-18.0103, -52.366) (-17.2714, -51.5215) (-16.1636, -51.0119) (-15.0416, -51.0002) (-13.8919, -50.9883) (-12.7469, -51.5006) (-11.9897, -52.366) knots -1 -1 -1 -1 -0.506107 -0.506107 -0.506107 0 0 0 0
  spline S459 degree 3 poles (-11.9897, -52.366) (-11.3663, -53.0785) (-11.0085, -54.0182) (-11.0002, -54.9649) (-10.9916, -55.935) (-11.3508, -56.9039) (-11.9897, -57.634) knots -1 -1 -1 -1 -0.506107 -0.506107 -0.506107 0 0 0 0
  spline S460 degree 3 poles (-11.9897, -47.634) (-12.7286, -48.4785) (-13.8364, -48.9881) (-14.9584, -48.9998) (-16.1081, -49.0117) (-17.2531, -48.4994) (-18.0103, -47.634) knots -1 -1 -1 -1 -0.506107 -0.506107 -0.506107 0 0 0 0
  spline S461 degree 3 poles (-18.0103, -47.634) (-18.6337, -46.9215) (-18.9915, -45.9818) (-18.9998, -45.0351) (-19.0084, -44.065) (-18.6492, -43.0961) (-18.0103, -42.366) knots -1 -1 -1 -1 -0.506107 -0.506107 -0.506107 0 0 0 0
  spline S462 degree 3 poles (-18.0103, -42.366) (-17.2714, -41.5215) (-16.1636, -41.0119) (-15.0416, -41.0002) (-13.8919, -40.9883) (-12.7469, -41.5006) (-11.9897, -42.366) knots -1 -1 -1 -1 -0.506107 -0.506107 -0.506107 0 0 0 0
  spline S463 degree 3 poles (-11.9897, -42.366) (-11.3663, -43.0785) (-11.0085, -44.0182) (-11.0002, -44.9649) (-10.9916, -45.935) (-11.3508, -46.9039) (-11.9897, -47.634) knots -1 -1 -1 -1 -0.506107 -0.506107 -0.506107 0 0 0 0
  spline S464 degree 3 poles (-11.9897, -37.634) (-12.7286, -38.4785) (-13.8364, -38.9881) (-14.9584, -38.9998) (-16.1081, -39.0117) (-17.2531, -38.4994) (-18.0103, -37.634) knots -1 -1 -1 -1 -0.506107 -0.506107 -0.506107 0 0 0 0
  spline S465 degree 3 poles (-18.0103, -37.634) (-18.6337, -36.9215) (-18.9915, -35.9818) (-18.9998, -35.0351) (-19.0084, -34.065) (-18.6492, -33.0961) (-18.0103, -32.366) knots -1 -1 -1 -1 -0.506107 -0.506107 -0.506107 0 0 0 0
  spline S466 degree 3 poles (-18.0103, -32.366) (-17.2714, -31.5215) (-16.1636, -31.0119) (-15.0416, -31.0002) (-13.8919, -30.9883) (-12.7469, -31.5006) (-11.9897, -32.366) knots -1 -1 -1 -1 -0.506107 -0.506107 -0.506107 0 0 0 0
  spline S467 degree 3 poles (-11.9897, -32.366) (-11.3663, -33.0785) (-11.0085, -34.0182) (-11.0002, -34.9649) (-10.9916, -35.935) (-11.3508, -36.9039) (-11.9897, -37.634) knots -1 -1 -1 -1 -0.506107 -0.506107 -0.506107 0 0 0 0
  spline S468 degree 3 poles (-11.9897, -27.634) (-12.7286, -28.4785) (-13.8364, -28.9881) (-14.9584, -28.9998) (-16.1081, -29.0117) (-17.2531, -28.4994) (-18.0103, -27.634) knots -1 -1 -1 -1 -0.506107 -0.506107 -0.506107 0 0 0 0
  spline S469 degree 3 poles (-18.0103, -27.634) (-18.6337, -26.9215) (-18.9915, -25.9818) (-18.9998, -25.0351) (-19.0084, -24.065) (-18.6492, -23.0961) (-18.0103, -22.366) knots -1 -1 -1 -1 -0.506107 -0.506107 -0.506107 0 0 0 0
  spline S470 degree 3 poles (-18.0103, -22.366) (-17.2714, -21.5215) (-16.1636, -21.0119) (-15.0416, -21.0002) (-13.8919, -20.9883) (-12.7469, -21.5006) (-11.9897, -22.366) knots -1 -1 -1 -1 -0.506107 -0.506107 -0.506107 0 0 0 0
  spline S471 degree 3 poles (-11.9897, -22.366) (-11.3663, -23.0785) (-11.0085, -24.0182) (-11.0002, -24.9649) (-10.9916, -25.935) (-11.3508, -26.9039) (-11.9897, -27.634) knots -1 -1 -1 -1 -0.506107 -0.506107 -0.506107 0 0 0 0
  spline S472 degree 3 poles (-11.9897, -17.634) (-12.7286, -18.4785) (-13.8364, -18.9881) (-14.9584, -18.9998) (-16.1081, -19.0117) (-17.2531, -18.4994) (-18.0103, -17.634) knots -1 -1 -1 -1 -0.506107 -0.506107 -0.506107 0 0 0 0
  spline S473 degree 3 poles (-18.0103, -17.634) (-18.6337, -16.9215) (-18.9915, -15.9818) (-18.9998, -15.0351) (-19.0084, -14.065) (-18.6492, -13.0961) (-18.0103, -12.366) knots -1 -1 -1 -1 -0.506107 -0.506107 -0.506107 0 0 0 0
  spline S474 degree 3 poles (-18.0103, -12.366) (-17.2714, -11.5215) (-16.1636, -11.0119) (-15.0416, -11.0002) (-13.8919, -10.9883) (-12.7469, -11.5006) (-11.9897, -12.366) knots -1 -1 -1 -1 -0.506107 -0.506107 -0.506107 0 0 0 0
  spline S475 degree 3 poles (-11.9897, -12.366) (-11.3663, -13.0785) (-11.0085, -14.0182) (-11.0002, -14.9649) (-10.9916, -15.935) (-11.3508, -16.9039) (-11.9897, -17.634) knots -1 -1 -1 -1 -0.506107 -0.506107 -0.506107 0 0 0 0
  spline S476 degree 3 poles (-11.9897, -7.634) (-12.7286, -8.4785) (-13.8364, -8.9881) (-14.9584, -8.9998) (-16.1081, -9.0117) (-17.2531, -8.4994) (-18.0103, -7.634) knots -1 -1 -1 -1 -0.506107 -0.506107 -0.506107 0 0 0 0
  spline S477 degree 3 poles (-18.0103, -7.634) (-18.6337, -6.9215) (-18.9915, -5.9818) (-18.9998, -5.0351) (-19.0084, -4.065) (-18.6492, -3.0961) (-18.0103, -2.366) knots -1 -1 -1 -1 -0.506107 -0.506107 -0.506107 0 0 0 0
  spline S478 degree 3 poles (-18.0103, -2.366) (-17.2714, -1.5215) (-16.1636, -1.0119) (-15.0416, -1.0002) (-13.8919, -0.9883) (-12.7469, -1.5006) (-11.9897, -2.366) knots -1 -1 -1 -1 -0.506107 -0.506107 -0.506107 0 0 0 0
  spline S479 degree 3 poles (-11.9897, -2.366) (-11.3663, -3.0785) (-11.0085, -4.0182) (-11.0002, -4.9649) (-10.9916, -5.935) (-11.3508, -6.9039) (-11.9897, -7.634) knots -1 -1 -1 -1 -0.506107 -0.506107 -0.506107 0 0 0 0
  spline S480 degree 3 poles (-1.9897, -77.634) (-2.7286, -78.4785) (-3.8364, -78.9881) (-4.9584, -78.9998) (-6.1081, -79.0117) (-7.2531, -78.4994) (-8.0103, -77.634) knots -1 -1 -1 -1 -0.506107 -0.506107 -0.506107 0 0 0 0
  spline S481 degree 3 poles (-8.0103, -77.634) (-8.6337, -76.9215) (-8.9915, -75.9818) (-8.9998, -75.0351) (-9.0084, -74.065) (-8.6492, -73.0961) (-8.0103, -72.366) knots -1 -1 -1 -1 -0.506107 -0.506107 -0.506107 0 0 0 0
  spline S482 degree 3 poles (-8.0103, -72.366) (-7.2714, -71.5215) (-6.1636, -71.0119) (-5.0416, -71.0002) (-3.8919, -70.9883) (-2.7469, -71.5006) (-1.9897, -72.366) knots -1 -1 -1 -1 -0.506107 -0.506107 -0.506107 0 0 0 0
  spline S483 degree 3 poles (-1.9897, -72.366) (-1.3663, -73.0785) (-1.0085, -74.0182) (-1.0002, -74.9649) (-0.9916, -75.935) (-1.3508, -76.9039) (-1.9897, -77.634) knots -1 -1 -1 -1 -0.506107 -0.506107 -0.506107 0 0 0 0
  spline S484 degree 3 poles (-1.9897, -67.634) (-2.7286, -68.4785) (-3.8364, -68.9881) (-4.9584, -68.9998) (-6.1081, -69.0117) (-7.2531, -68.4994) (-8.0103, -67.634) knots -1 -1 -1 -1 -0.506107 -0.506107 -0.506107 0 0 0 0
  spline S485 degree 3 poles (-8.0103, -67.634) (-8.6337, -66.9215) (-8.9915, -65.9818) (-8.9998, -65.0351) (-9.0084, -64.065) (-8.6492, -63.0961) (-8.0103, -62.366) knots -1 -1 -1 -1 -0.506107 -0.506107 -0.506107 0 0 0 0
  spline S486 degree 3 poles (-8.0103, -62.366) (-7.2714, -61.5215) (-6.1636, -61.0119) (-5.0416, -61.0002) (-3.8919, -60.9883) (-2.7469, -61.5006) (-1.9897, -62.366) knots -1 -1 -1 -1 -0.506107 -0.506107 -0.506107 0 0 0 0
  spline S487 degree 3 poles (-1.9897, -62.366) (-1.3663, -63.0785) (-1.0085, -64.0182) (-1.0002, -64.9649) (-0.9916, -65.935) (-1.3508, -66.9039) (-1.9897, -67.634) knots -1 -1 -1 -1 -0.506107 -0.506107 -0.506107 0 0 0 0
  spline S488 degree 3 poles (-1.9897, -57.634) (-2.7286, -58.4785) (-3.8364, -58.9881) (-4.9584, -58.9998) (-6.1081, -59.0117) (-7.2531, -58.4994) (-8.0103, -57.634) knots -1 -1 -1 -1 -0.506107 -0.506107 -0.506107 0 0 0 0
  spline S489 degree 3 poles (-8.0103, -57.634) (-8.6337, -56.9215) (-8.9915, -55.9818) (-8.9998, -55.0351) (-9.0084, -54.065) (-8.6492, -53.0961) (-8.0103, -52.366) knots -1 -1 -1 -1 -0.506107 -0.506107 -0.506107 0 0 0 0
  spline S490 degree 3 poles (-8.0103, -52.366) (-7.2714, -51.5215) (-6.1636, -51.0119) (-5.0416, -51.0002) (-3.8919, -50.9883) (-2.7469, -51.5006) (-1.9897, -52.366) knots -1 -1 -1 -1 -0.506107 -0.506107 -0.506107 0 0 0 0
  spline S491 degree 3 poles (-1.9897, -52.366) (-1.3663, -53.0785) (-1.0085, -54.0182) (-1.0002, -54.9649) (-0.9916, -55.935) (-1.3508, -56.9039) (-1.9897, -57.634) knots -1 -1 -1 -1 -0.506107 -0.506107 -0.506107 0 0 0 0
  spline S492 degree 3 poles (-1.9897, -47.634) (-2.7286, -48.4785) (-3.8364, -48.9881) (-4.9584, -48.9998) (-6.1081, -49.0117) (-7.2531, -48.4994) (-8.0103, -47.634) knots -1 -1 -1 -1 -0.506107 -0.506107 -0.506107 0 0 0 0
  spline S493 degree 3 poles (-8.0103, -47.634) (-8.6337, -46.9215) (-8.9915, -45.9818) (-8.9998, -45.0351) (-9.0084, -44.065) (-8.6492, -43.0961) (-8.0103, -42.366) knots -1 -1 -1 -1 -0.506107 -0.506107 -0.506107 0 0 0 0
  spline S494 degree 3 poles (-8.0103, -42.366) (-7.2714, -41.5215) (-6.1636, -41.0119) (-5.0416, -41.0002) (-3.8919, -40.9883) (-2.7469, -41.5006) (-1.9897, -42.366) knots -1 -1 -1 -1 -0.506107 -0.506107 -0.506107 0 0 0 0
  spline S495 degree 3 poles (-1.9897, -42.366) (-1.3663, -43.0785) (-1.0085, -44.0182) (-1.0002, -44.9649) (-0.9916, -45.935) (-1.3508, -46.9039) (-1.9897, -47.634) knots -1 -1 -1 -1 -0.506107 -0.506107 -0.506107 0 0 0 0
  spline S496 degree 3 poles (-1.9897, -37.634) (-2.7286, -38.4785) (-3.8364, -38.9881) (-4.9584, -38.9998) (-6.1081, -39.0117) (-7.2531, -38.4994) (-8.0103, -37.634) knots -1 -1 -1 -1 -0.506107 -0.506107 -0.506107 0 0 0 0
  spline S497 degree 3 poles (-8.0103, -37.634) (-8.6337, -36.9215) (-8.9915, -35.9818) (-8.9998, -35.0351) (-9.0084, -34.065) (-8.6492, -33.0961) (-8.0103, -32.366) knots -1 -1 -1 -1 -0.506107 -0.506107 -0.506107 0 0 0 0
  spline S498 degree 3 poles (-8.0103, -32.366) (-7.2714, -31.5215) (-6.1636, -31.0119) (-5.0416, -31.0002) (-3.8919, -30.9883) (-2.7469, -31.5006) (-1.9897, -32.366) knots -1 -1 -1 -1 -0.506107 -0.506107 -0.506107 0 0 0 0
  spline S499 degree 3 poles (-1.9897, -32.366) (-1.3663, -33.0785) (-1.0085, -34.0182) (-1.0002, -34.9649) (-0.9916, -35.935) (-1.3508, -36.9039) (-1.9897, -37.634) knots -1 -1 -1 -1 -0.506107 -0.506107 -0.506107 0 0 0 0
  spline S500 degree 3 poles (-1.9897, -27.634) (-2.7286, -28.4785) (-3.8364, -28.9881) (-4.9584, -28.9998) (-6.1081, -29.0117) (-7.2531, -28.4994) (-8.0103, -27.634) knots -1 -1 -1 -1 -0.506107 -0.506107 -0.506107 0 0 0 0
  spline S501 degree 3 poles (-8.0103, -27.634) (-8.6337, -26.9215) (-8.9915, -25.9818) (-8.9998, -25.0351) (-9.0084, -24.065) (-8.6492, -23.0961) (-8.0103, -22.366) knots -1 -1 -1 -1 -0.506107 -0.506107 -0.506107 0 0 0 0
  spline S502 degree 3 poles (-8.0103, -22.366) (-7.2714, -21.5215) (-6.1636, -21.0119) (-5.0416, -21.0002) (-3.8919, -20.9883) (-2.7469, -21.5006) (-1.9897, -22.366) knots -1 -1 -1 -1 -0.506107 -0.506107 -0.506107 0 0 0 0
  spline S503 degree 3 poles (-1.9897, -22.366) (-1.3663, -23.0785) (-1.0085, -24.0182) (-1.0002, -24.9649) (-0.9916, -25.935) (-1.3508, -26.9039) (-1.9897, -27.634) knots -1 -1 -1 -1 -0.506107 -0.506107 -0.506107 0 0 0 0
  spline S504 degree 3 poles (-1.9897, -17.634) (-2.7286, -18.4785) (-3.8364, -18.9881) (-4.9584, -18.9998) (-6.1081, -19.0117) (-7.2531, -18.4994) (-8.0103, -17.634) knots -1 -1 -1 -1 -0.506107 -0.506107 -0.506107 0 0 0 0
  spline S505 degree 3 poles (-8.0103, -17.634) (-8.6337, -16.9215) (-8.9915, -15.9818) (-8.9998, -15.0351) (-9.0084, -14.065) (-8.6492, -13.0961) (-8.0103, -12.366) knots -1 -1 -1 -1 -0.506107 -0.506107 -0.506107 0 0 0 0
  spline S506 degree 3 poles (-8.0103, -12.366) (-7.2714, -11.5215) (-6.1636, -11.0119) (-5.0416, -11.0002) (-3.8919, -10.9883) (-2.7469, -11.5006) (-1.9897, -12.366) knots -1 -1 -1 -1 -0.506107 -0.506107 -0.506107 0 0 0 0
  spline S507 degree 3 poles (-1.9897, -12.366) (-1.3663, -13.0785) (-1.0085, -14.0182) (-1.0002, -14.9649) (-0.9916, -15.935) (-1.3508, -16.9039) (-1.9897, -17.634) knots -1 -1 -1 -1 -0.506107 -0.506107 -0.506107 0 0 0 0
  spline S508 degree 3 poles (-1.9897, -7.634) (-2.7286, -8.4785) (-3.8364, -8.9881) (-4.9584, -8.9998) (-6.1081, -9.0117) (-7.2531, -8.4994) (-8.0103, -7.634) knots -1 -1 -1 -1 -0.506107 -0.506107 -0.506107 0 0 0 0
  spline S509 degree 3 poles (-8.0103, -7.634) (-8.6337, -6.9215) (-8.9915, -5.9818) (-8.9998, -5.0351) (-9.0084, -4.065) (-8.6492, -3.0961) (-8.0103, -2.366) knots -1 -1 -1 -1 -0.506107 -0.506107 -0.506107 0 0 0 0
  spline S510 degree 3 poles (-8.0103, -2.366) (-7.2714, -1.5215) (-6.1636, -1.0119) (-5.0416, -1.0002) (-3.8919, -0.9883) (-2.7469, -1.5006) (-1.9897, -2.366) knots -1 -1 -1 -1 -0.506107 -0.506107 -0.506107 0 0 0 0
  spline S511 degree 3 poles (-1.9897, -2.366) (-1.3663, -3.0785) (-1.0085, -4.0182) (-1.0002, -4.9649) (-0.9916, -5.935) (-1.3508, -6.9039) (-1.9897, -7.634) knots -1 -1 -1 -1 -0.506107 -0.506107 -0.506107 0 0 0 0
  line L0 (1, 1) -> (-161, 1)
  line L1 (-161, 1) -> (-161, -81)
  line L2 (-161, -81) -> (1, -81)
  line L3 (1, -81) -> (1, 1)
  line L4 (1, -81) -> (-161, -81)
  line L5 (-161, -81) -> (-161, 1)
  line L6 (-161, 1) -> (1, 1)
  line L7 (1, 1) -> (1, -81)
  constraint horizontal L4